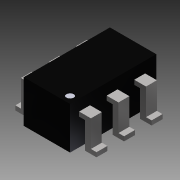
# Autodesk Inventor part: 74LVC2G14 Dual Inverter
Saved by Autodesk Inventor 2015 (Build 190159000, 159)
## iProperties
Created: 2016-01-19
Part Number: 74LVC2G14 Dual Inverter
Material: Generic
Document SubType Name: Modeling
Designer: Kyle
Density: 1 g/cm^3
Appearance: Default
Author: Kyle
Autodesk Inventor part; units mm, degrees
ref_plane "YZ Plane" through (0, 0, 0) normal (1, 0, 0) x (0, 1, 0)
ref_plane "XZ Plane" through (0, 0, 0) normal (0, 1, 0) x (-1, 0, 0)
ref_plane "XY Plane" through (0, 0, 0) normal (0, 0, 1) x (1, 0, 0)
sketch "Sketch1" plane through (0, 0, 0) normal (0, 0, 1) x (1, 0, 0)
  line L0 (0, 0) -> (1.6002, 0)
  line L1 (1.6002, 0) -> (1.6002, 1.4503)
  line L2 (1.6002, 1.4503) -> (0, 1.4503)
  line L3 (0, 1.4503) -> (0, 0)
  dimension "d0" = 1.6002
  dimension "d1" = 1.4503
  constraints: 8 end point, 2 parallel, 1 horizontal, 1 perpendicular
  measures "d0" distance of L1.end L2.end
  measures "d1" distance of L0.end L1.end
extrude "Extrusion1" add sketch "Sketch1" along normal blind 2.9743
sketch "Sketch2" plane through (1.6002, 0, 0) normal (1, 0, 0) x (0, 0, -1)
  line L0 (-2.6619, 1.0693) -> (-2.286, 1.0693)
  line L1 (-2.286, 1.0693) -> (-2.286, 0.9169)
  line L2 (-2.286, 0.9169) -> (-2.6619, 0.9169)
  line L3 (-2.6619, 0.9169) -> (-2.6619, 1.0693)
  line L4 (0, 1.4503) -> (-2.9743, 1.4503) projected
  line L5 (-2.9743, 0) -> (-2.9743, 1.4503) projected
  line L6 (-1.712, 1.0693) -> (-1.336, 1.0693)
  line L7 (-1.336, 1.0693) -> (-1.336, 0.9169)
  line L8 (-1.336, 0.9169) -> (-1.712, 0.9169)
  line L9 (-1.712, 0.9169) -> (-1.712, 1.0693)
  line L10 (-0.762, 1.0693) -> (-0.3861, 1.0693)
  line L11 (-0.3861, 1.0693) -> (-0.3861, 0.9169)
  line L12 (-0.3861, 0.9169) -> (-0.762, 0.9169)
  line L13 (-0.762, 0.9169) -> (-0.762, 1.0693)
  point P0 (0, 0)
  dimension "d4" = 0.1524
  dimension "d5" = 0.3759
  dimension "d6" = 0.381
  dimension "d7" = 0.3124
  dimension "d10" = 0.95
  constraints: 24 end point, 2 horizontal, 2 parallel, 1 perpendicular, 16 other
  measures "d4" distance of L2.end L0.start
  measures "d5" distance of L0.start L0.end
  measures "d6" distance between parallel lines of L4 L0
  measures "d7" distance between parallel lines of L5 L3
  measures "d10" distance of L0.start L6.start
extrude "Extrusion2" add sketch "Sketch2" along normal blind 0.254
extrude "Extrusion3" add sketch "Sketch2" against normal blind 1.8542
sketch "Sketch3" plane through (1.8542, 0, 0) normal (1, 0, 0) x (0, 0, -1)
  line L0 (-2.6619, 0.9169) -> (-2.286, 0.9169)
  line L1 (-2.286, 0.9169) -> (-2.286, 1.0693)
  line L2 (-2.286, 1.0693) -> (-2.6619, 1.0693)
  line L3 (-2.6619, 1.0693) -> (-2.6619, 0.9169)
  line L4 (-1.712, 0.9169) -> (-1.336, 0.9169)
  line L5 (-1.336, 0.9169) -> (-1.336, 1.0693)
  line L6 (-1.336, 1.0693) -> (-1.712, 1.0693)
  line L7 (-1.712, 1.0693) -> (-1.712, 0.9169)
  line L8 (-0.762, 0.9169) -> (-0.3861, 0.9169)
  line L9 (-0.3861, 0.9169) -> (-0.3861, 1.0693)
  line L10 (-0.3861, 1.0693) -> (-0.762, 1.0693)
  line L11 (-0.762, 1.0693) -> (-0.762, 0.9169)
  point P0 (0, 0)
  constraints: 24 end point, 6 parallel, 3 horizontal, 3 perpendicular
extrude "Extrusion4" add sketch "Sketch3" along normal blind 0.1524
sketch "Sketch4" plane through (-0.254, 0, 0) normal (-1, 0, 0) x (0, 0, 1)
  line L0 (2.286, 1.0693) -> (2.6619, 1.0693)
  line L1 (2.6619, 1.0693) -> (2.6619, 0.9169)
  line L2 (2.6619, 0.9169) -> (2.286, 0.9169)
  line L3 (2.286, 0.9169) -> (2.286, 1.0693)
  line L4 (1.712, 1.0693) -> (1.336, 1.0693)
  line L5 (1.336, 1.0693) -> (1.336, 0.9169)
  line L6 (1.336, 0.9169) -> (1.712, 0.9169)
  line L7 (1.712, 0.9169) -> (1.712, 1.0693)
  line L8 (0.762, 1.0693) -> (0.3861, 1.0693)
  line L9 (0.3861, 1.0693) -> (0.3861, 0.9169)
  line L10 (0.3861, 0.9169) -> (0.762, 0.9169)
  line L11 (0.762, 0.9169) -> (0.762, 1.0693)
  point P0 (0, 0)
  constraints: 24 end point, 6 parallel, 3 horizontal, 3 perpendicular
extrude "Extrusion5" add sketch "Sketch4" along normal blind 0.1524
sketch "Sketch5" plane through (0, 0.9169, 2.286) normal (0, -1, 0) x (1, 0, 0)
  line L0 (0, 0) -> (-0.4064, 0) projected
  line L1 (-0.4064, 0.3759) -> (-0.2032, 0.3759)
  line L2 (-0.2032, 0.3759) -> (-0.2032, 0)
  line L3 (-0.2032, 0) -> (-0.4064, 0)
  line L4 (-0.4064, 0) -> (-0.4064, 0.3759)
  line L5 (0, -0.95) -> (-0.4064, -0.95) projected
  line L6 (-0.4064, -0.574) -> (-0.2032, -0.574)
  line L7 (-0.2032, -0.574) -> (-0.2032, -0.95)
  line L8 (-0.2032, -0.95) -> (-0.4064, -0.95)
  line L9 (-0.4064, -0.95) -> (-0.4064, -0.574)
  line L10 (0, -1.8999) -> (-0.4064, -1.8999) projected
  line L11 (-0.4064, -1.524) -> (-0.2032, -1.524)
  line L12 (-0.2032, -1.524) -> (-0.2032, -1.8999)
  line L13 (-0.2032, -1.8999) -> (-0.4064, -1.8999)
  line L14 (-0.4064, -1.8999) -> (-0.4064, -1.524)
  line L15 (1.6002, 0) -> (2.0066, 0) projected
  line L16 (2.0066, 0.3759) -> (1.8034, 0.3759)
  line L17 (1.8034, 0.3759) -> (1.8034, 0)
  line L18 (1.8034, 0) -> (2.0066, 0)
  line L19 (2.0066, 0) -> (2.0066, 0.3759)
  line L20 (2.0066, -0.574) -> (1.8034, -0.574)
  line L21 (1.8034, -0.574) -> (1.8034, -0.95)
  line L22 (1.8034, -0.95) -> (2.0066, -0.95)
  line L23 (2.0066, -0.95) -> (2.0066, -0.574)
  line L24 (1.6002, -1.8999) -> (2.0066, -1.8999) projected
  line L25 (2.0066, -1.524) -> (1.8034, -1.524)
  line L26 (1.8034, -1.524) -> (1.8034, -1.8999)
  line L27 (1.8034, -1.8999) -> (2.0066, -1.8999)
  line L28 (2.0066, -1.8999) -> (2.0066, -1.524)
  point P0 (0, -2.286)
  constraints: 48 end point, 12 parallel, 6 horizontal, 6 perpendicular, 5 midpoint, 2 point on line
extrude "Extrusion6" add sketch "Sketch5" along normal blind 0.9144
sketch "Sketch6" plane through (2.0066, 0, 0) normal (1, 0, 0) x (0, 0, -1)
  line L0 (-2.286, 0.9169) -> (-2.286, 0.0025) projected
  line L1 (-2.6619, 0.0025) -> (-2.286, 0.0025)
  line L2 (-2.286, 0.0025) -> (-2.286, 0.1549)
  line L3 (-2.286, 0.1549) -> (-2.6619, 0.1549)
  line L4 (-2.6619, 0.1549) -> (-2.6619, 0.0025)
  line L5 (-1.336, 1.0693) -> (-1.336, 0.0025) projected
  line L6 (-1.712, 0.0025) -> (-1.336, 0.0025)
  line L7 (-1.336, 0.0025) -> (-1.336, 0.1549)
  line L8 (-1.336, 0.1549) -> (-1.712, 0.1549)
  line L9 (-1.712, 0.1549) -> (-1.712, 0.0025)
  line L10 (-0.3861, 1.0693) -> (-0.3861, 0.0025) projected
  line L11 (-0.762, 0.0025) -> (-0.3861, 0.0025)
  line L12 (-0.3861, 0.0025) -> (-0.3861, 0.1549)
  line L13 (-0.3861, 0.1549) -> (-0.762, 0.1549)
  line L14 (-0.762, 0.1549) -> (-0.762, 0.0025)
  point P0 (0, 0)
  dimension "d25" = 0.1524
  constraints: 24 end point, 6 parallel, 4 point on line, 3 horizontal, 3 perpendicular
  measures "d25" distance of L3.end L1.start
extrude "Extrusion7" add sketch "Sketch6" along normal blind 0.193
sketch "Sketch7" plane through (-0.4064, 0, 0) normal (-1, 0, 0) x (0, 0, 1)
  line L0 (2.286, 0.0025) -> (2.6619, 0.0025)
  line L1 (2.6619, 0.0025) -> (2.6619, 0.1549)
  line L2 (2.6619, 0.1549) -> (2.286, 0.1549)
  line L3 (2.286, 0.1549) -> (2.286, 0.0025)
  line L4 (1.712, 0.0025) -> (1.336, 0.0025)
  line L5 (1.336, 0.0025) -> (1.336, 0.1549)
  line L6 (1.336, 0.1549) -> (1.712, 0.1549)
  line L7 (1.712, 0.1549) -> (1.712, 0.0025)
  line L8 (0.762, 0.0025) -> (0.3861, 0.0025)
  line L9 (0.3861, 0.0025) -> (0.3861, 0.1549)
  line L10 (0.3861, 0.1549) -> (0.762, 0.1549)
  line L11 (0.762, 0.1549) -> (0.762, 0.0025)
  point P0 (0, 0)
  constraints: 24 end point, 6 parallel, 3 horizontal, 3 perpendicular
extrude "Extrusion8" add sketch "Sketch7" along normal blind 0.193
sketch "Sketch8" plane through (0, 1.4503, 0) normal (0, 1, 0) x (1, 0, 0)
  circle A0 centre (1.3462, -2.7203) radius 0.127
  line L0 (1.6002, 0) -> (1.6002, -2.9743) projected
  line L1 (1.6002, -2.9743) -> (0, -2.9743) projected
  point P0 (0, 0)
  dimension "d30" = 0.254
  dimension "d31" = 0.254
  dimension "d32" = 0.254
  constraints: 1 centre point
  measures "d30" diameter of A0
  measures "d31" distance from line of L0 A0.centre
  measures "d32" distance from line of L1 A0.centre
extrude "Extrusion9" cut sketch "Sketch8" against normal blind 0.0254
body "Solid1"
